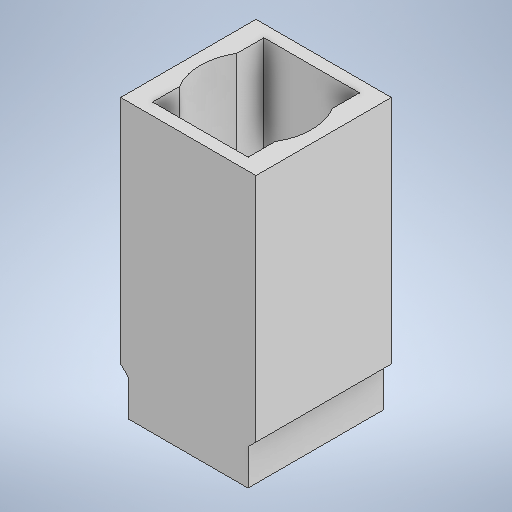
# Autodesk Inventor part: BambuLabVolcanoNozzle_silicon_innerpart2
Saved by Autodesk Inventor 2025.2 (Build 292293000, 293)
## iProperties
Created: 2025-02-18
Part Number: BambuLabVolcanoNozzle_silicon_innerpart2
Material: Generisch
Document SubType Name: Modeling
Designer: FrankFlorian
Density: 1 g/cm^3
Appearance: Vorgabe
Author: FrankFlorian
Autodesk Inventor part; units mm, degrees
ref_plane "YZ Plane" through (0, 0, 0) normal (1, 0, 0) x (0, 1, 0)
ref_plane "XZ Plane" through (0, 0, 0) normal (0, 1, 0) x (-1, 0, 0)
ref_plane "XY Plane" through (0, 0, 0) normal (0, 0, 1) x (1, 0, 0)
sketch "Skizze1" plane through (0, 0, 0) normal (0, 0, 1) x (1, 0, 0)
  line L0 (-7.5, 8.5) -> (7.5, 8.5)
  line L1 (7.5, 8.5) -> (7.5, -8.5)
  line L2 (7.5, -8.5) -> (-7.5, -8.5)
  line L3 (-7.5, -8.5) -> (-7.5, 8.5)
  line L4 (-7.5, 8.5) -> (7.5, -8.5) construction
  line L5 (7.5, 8.5) -> (-7.5, -8.5) construction
  circle A0 centre (0, 0) radius 1.4
  dimension "d0" = 15
  dimension "d1" = 2.8
  dimension "d5" = 17
  constraints: 12 end point, 2 midpoint, 2 parallel, 1 centre point, 1 coincident, 1 horizontal, 1 perpendicular
  measures "d0" distance of L1.end L2.end
  measures "d1" diameter of A0
  measures "d5" distance of L0.end L1.end
extrude "Extrusion1" add sketch "Skizze1" along normal blind 2
sketch "Skizze2" plane through (0, 0, 2) normal (0, 0, 1) x (1, 0, 0)
  circle A0 centre (0, 0) radius 5.5
  line L0 (-7.5, -8.5) -> (7.5, -8.5) projected
  line L1 (-7.5, 8.5) -> (7.5, 8.5)
  line L2 (7.5, 8.5) -> (7.5, -8.5)
  line L3 (7.5, -8.5) -> (-7.5, -8.5)
  line L4 (-7.5, -8.5) -> (-7.5, 8.5)
  circle A1 centre (0, 0) radius 1.4 projected
  line L5 (-7.5, 8.5) -> (7.5, -8.5) construction
  line L6 (7.5, 8.5) -> (-7.5, -8.5) construction
  dimension "d4" = 11
  constraints: 12 end point, 2 midpoint, 2 parallel, 1 centre point, 1 coincident, 1 horizontal, 1 perpendicular
  measures "d4" diameter of A0
extrude "Extrusion2" add sketch "Skizze2" along normal blind 3.5 contours L4 L1 L2 L0
sketch "Skizze3" plane through (0, 0, 5.5) normal (0, 0, 1) x (1, 0, 0)
  circle A0 centre (0, 0) radius 7
  line L0 (-8.5, 8.5) -> (8.5, 8.5)
  line L1 (8.5, 8.5) -> (8.5, -8.5)
  line L2 (8.5, -8.5) -> (-8.5, -8.5)
  line L3 (-8.5, -8.5) -> (-8.5, 8.5)
  line L4 (-8.5, 8.5) -> (8.5, -8.5) construction
  line L5 (8.5, 8.5) -> (-8.5, -8.5) construction
  dimension "d8" = 14
  dimension "d9" = 17
  constraints: 12 end point, 2 midpoint, 2 parallel, 1 centre point, 1 coincident, 1 horizontal, 1 perpendicular
  measures "d8" diameter of A0
  measures "d9" distance of L1.end L2.end
extrude "Extrusion3" add sketch "Skizze3" along normal blind 10
sketch "Skizze4" plane through (0, 0, 15.5) normal (0, 0, 1) x (1, 0, 0)
  line L0 (-6, 7) -> (6, 7)
  line L1 (6, 7) -> (6, -7)
  line L2 (6, -7) -> (-6, -7)
  line L3 (-6, -7) -> (-6, 7)
  line L4 (-6, 7) -> (6, -7) construction
  line L5 (6, 7) -> (-6, -7) construction
  line L6 (-8.5, -8.5) -> (8.5, -8.5) projected
  line L7 (-8.5, 8.5) -> (8.5, 8.5)
  line L8 (8.5, 8.5) -> (8.5, -8.5)
  line L9 (8.5, -8.5) -> (-8.5, -8.5)
  line L10 (-8.5, -8.5) -> (-8.5, 8.5)
  line L11 (-8.5, 8.5) -> (8.5, -8.5) construction
  line L12 (8.5, 8.5) -> (-8.5, -8.5) construction
  circle A0 centre (0, 0) radius 7
  point P0 (6, 3.6056)
  point P1 (6, -3.6056)
  point P2 (-6, -3.6056)
  point P3 (-6, 3.6056)
  dimension "d12" = 12
  dimension "d13" = 14
  dimension "d19" = 17
  constraints: 24 end point, 4 midpoint, 4 parallel, 2 horizontal, 2 perpendicular, 1 centre point, 1 coincident
  measures "d12" distance of L1.end L2.end
  measures "d13" distance of L0.end L1.end
  measures "d19" distance of L9.end L7.start
extrude "Extrusion4" add sketch "Skizze4" along normal blind 19
chamfer "Fasen1" distance 1 angle 45 2 edges at (7.5, 0, 5.5) (-7.5, 0, 5.5)
sketch "Skizze5" plane through (-8.5, -8.5, 34.5) normal (-1, 0, 0) x (0, 0, 1)
  point P0 (-34.5, 8.5)
